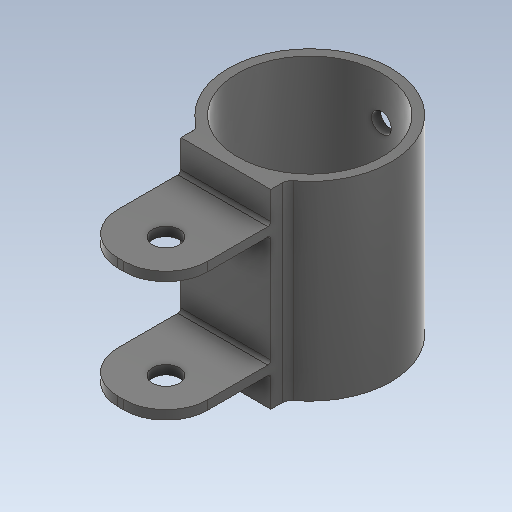
# Autodesk Inventor part: Hanger_Clamp
Saved by Autodesk Inventor 2020 (Build 240168000, 168)
## iProperties
Created: 2021-07-08
Part Number: Hanger_Clamp
Material: Steel, Carbon
Document SubType Name: Modeling
Designer: Simon.Alvarez
Density: 7.85 g/cm^3
Appearance: Semi-Polished
Author: Simon.Alvarez
Autodesk Inventor part; units mm, degrees
ref_plane "YZ Plane" through (0, 0, 0) normal (1, 0, 0) x (0, 1, 0)
ref_plane "XZ Plane" through (0, 0, 0) normal (0, 1, 0) x (-1, 0, 0)
ref_plane "XY Plane" through (0, 0, 0) normal (0, 0, 1) x (1, 0, 0)
sketch "Sketch1" plane through (0, 0, 0) normal (0, 1, 0) x (-1, 0, 0)
  circle A0 centre (0, 0) radius 24.125
  arc A1 (-16.2075, 21.7505) -> (16.2075, 21.7505) centre (0, 0) ccw
  line L0 (15, 28) -> (-15, 28)
  line L1 (-15, 28) -> (-15, 25.1875)
  line L2 (15, 24.1561) -> (15, 28)
  line L3 (15, 28) -> (-15, 25.1875) construction
  line L4 (-15, 28) -> (15, 24.7857) construction
  line L5 (-15, 25.1875) -> (-15, 24.1561)
  arc A2 (15, 24.1561) -> (16.2075, 21.7505) centre (18, 24.1561) ccw
  arc A3 (-16.2075, 21.7505) -> (-15, 24.1561) centre (-18, 24.1561) ccw
  point P0 (-1, 26.5)
  point P1 (0, 26.3929)
  point P2 (15, 22.6001)
  point P3 (-15, 22.6001)
  dimension "d0" = 48.25
  dimension "d2" = 3
  dimension "d4" = 30
  dimension "d6" = 28
  dimension "d7" = 3
  constraints: 12 end point, 8 point on circle, 5 point on line, 4 centre point, 4 tangent, 1 coincident, 1 equal radius, 1 horizontal, 1 midpoint, 1 parallel, 1 perpendicular, 1 vertical, 1 vertical alignment
  measures "d0" diameter of A0
  measures "d2" radial gap between concentric circles of A0 A1
  measures "d4" distance of L0.start L0.end
  measures "d6" distance from line of L0 point (0, 0)
  measures "d7" radius of A2
extrude "Extrusion1" add sketch "Sketch1" along normal blind 63.5
sketch "Sketch2" plane through (-15, 0, 28) normal (0, 0, 1) x (1, 0, 0)
  line L0 (30, 0) -> (30, 63.5) projected
  line L1 (0, 50.25) -> (30, 50.25)
  line L2 (30, 50.25) -> (30, 53.25)
  line L3 (30, 53.25) -> (0, 53.25)
  line L4 (0, 53.25) -> (0, 50.25)
  line L5 (0, 50.25) -> (30, 53.25) construction
  line L6 (30, 50.25) -> (0, 53.25) construction
  line L7 (0, 10.25) -> (30, 10.25)
  line L8 (30, 10.25) -> (30, 13.25)
  line L9 (30, 13.25) -> (0, 13.25)
  line L10 (0, 13.25) -> (0, 10.25)
  line L11 (0, 10.25) -> (30, 13.25) construction
  line L12 (30, 10.25) -> (0, 13.25) construction
  line L13 (0, 0) -> (0, 63.5) projected
  line L14 (0, 31.75) -> (30, 31.75) construction
  point P0 (15, 0)
  point P1 (15, 51.75)
  point P2 (15, 11.75)
  dimension "d10" = 3
  dimension "d11" = 3
  dimension "d12" = 40
  dimension "d13" = 20
  dimension "d34" = 30
  dimension "d35" = 30
  constraints: 26 end point, 6 midpoint, 4 parallel, 2 horizontal, 2 perpendicular, 2 point on line
  measures "d10" distance of L9.end L7.start
  measures "d11" distance of L3.end L1.start
  measures "d12" distance of point (15, 11.75) point (15, 51.75)
  measures "d13" distance from line of L14 point (15, 51.75)
  measures "d34" distance of L2.end L3.end
  measures "d35" distance of L7.start L7.end
extrude "Extrusion2" add sketch "Sketch2" along normal blind 35 contours L7 L10 L9 L0 | L1 L4 L3 L0
fillet "Fillet1" radius 14 4 edges at (-15, 51.75, 63) (15, 11.75, 63) (15, 51.75, 63) (-15, 11.75, 63)
sketch "Sketch3" plane through (-15, 53.25, 28) normal (0, 1, 0) x (1, 0, 0)
  arc A0 (0, -21) -> (30, -21) centre (16, -21) ccw projected
  point P0 (15, 28)
  constraints: 1 coincident, 1 other
hole "Hole1" at (1, 53.25, 49) direction (0, -1, 0) diameter 9 end through all clearance for "Flat Head Machine Screw" size "M8" standard "Ansi Metric M Profile"
fillet "Fillet2" radius 1 4 edges at (0, 53.25, 28) (0, 50.25, 28) (0, 13.25, 28) (0, 10.25, 28)
sketch "Sketch4" plane through (0, 0, 0) normal (0, 0, 1) x (1, 0, 0)
  line L0 (16.2075, 0) -> (16.2075, 63.5) projected
  line L1 (16.2075, 31.75) -> (-16.2075, 31.75)
  line L2 (-16.2075, 0) -> (-16.2075, 63.5) projected
  point P0 (0, 0)
  point P1 (0, 49.25)
  point P2 (0, 14.25)
  point P3 (0, 31.75)
  dimension "d25" = 17.5
  dimension "d26" = 17.5
  constraints: 3 midpoint, 2 end point, 1 vertical alignment
  measures "d25" distance from line of L1 point (0, 49.25)
  measures "d26" distance of point (0, 14.25) point (0, 31.75)
hole "Hole2" at (0, 49.25, 0) at (0, 14.25, 0) direction (0, 0, -1) diameter 6.6 end through all clearance for "Flat Head Machine Screw" size "M6" standard "Ansi Metric M Profile"
equation "\"d13\" = 0.5 * d12"
equation "\"d25\" = 0.5 * Clamp_Bolt_Space"
equation "\"d26\" = d25"
equation "\"Clamp_Bolt_Space\" = 35"
body "Solid1"
